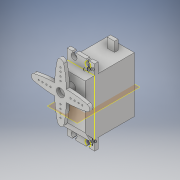
# Autodesk Inventor part: Hew Motor
Saved by Autodesk Inventor 2017 (Build 210142000, 142)
## iProperties
Created: 2016-09-26
Part Number: Hew Motor
Material: Generic
Document SubType Name: Modeling
Designer: situh
Density: 1 g/cm^3
Appearance: Default
Author: situh
Autodesk Inventor part; units mm, degrees
ref_plane "YZ Plane" through (0, 0, 0) normal (1, 0, 0) x (0, 1, 0)
ref_plane "XZ Plane" through (0, 0, 0) normal (0, 1, 0) x (-1, 0, 0)
ref_plane "XY Plane" through (0, 0, 0) normal (0, 0, 1) x (1, 0, 0)
sketch "Sketch1" plane through (0, 0, 0) normal (0, 0, 1) x (1, 0, 0)
  line L0 (-0.8096, 19.4036) -> (19.1904, 19.4036)
  line L1 (19.1904, 19.4036) -> (19.1904, -21.0964)
  line L2 (19.1904, -21.0964) -> (-0.8096, -21.0964)
  line L3 (-0.8096, -21.0964) -> (-0.8096, 19.4036)
  point P0 (0, 0)
  dimension "d0" = 40.5
  dimension "d1" = 20
  constraints: 8 end point, 2 parallel, 1 horizontal, 1 perpendicular
  measures "d0" distance of L0.end L1.end
  measures "d1" distance of L0.start L0.end
extrude "Extrusion1" add sketch "Sketch1" along normal blind 35.9918
sketch "Sketch2" plane through (0, 0, 35.9918) normal (0, 0, 1) x (1, 0, 0)
  circle A0 centre (9.2336, 11.0968) radius 2.9464
  point P0 (0, 0)
  point P1 (-0.8096, -21.0964)
  point P2 (19.1904, -21.0964)
  dimension "d5" = 5.8928
  constraints: 1 centre point
  measures "d5" diameter of A0
extrude "Extrusion2" add sketch "Sketch2" along normal blind 5.6896
sketch "Sketch3" plane through (-0.8096, -21.0964, 0) normal (0, -1, 0) x (1, 0, 0)
  line L0 (0, 0) -> (0, 35.9918) projected
  line L1 (20, 0) -> (20, 35.9918) projected
  line L2 (0, 29.1) -> (20, 29.1)
  line L3 (20, 29.1) -> (20, 26.6)
  line L4 (20, 26.6) -> (0, 26.6)
  line L5 (0, 26.6) -> (0, 29.1)
  point P0 (0.8096, 0)
  dimension "d9" = 2.5
  dimension "d48" = 26.6
  constraints: 8 end point, 2 parallel, 2 point on line, 1 horizontal, 1 perpendicular
  measures "d9" distance of L4.end L2.start
  measures "d48" distance of L3.end L1.start
extrude "Extrusion3" add sketch "Sketch3" along normal blind 7.4168
ref_plane "Work Plane1" through (-0.8096, -0.8464, 35.9918) normal (0, 1, 0) x (1, 0, 0)
sketch "Sketch5" plane through (-0.8096, -21.0964, 29.1) normal (0, 0, 1) x (1, 0, 0)
  arc A0 (5.7377, -6.6011) -> (4.2533, -6.5978) centre (5, -4.572) ccw
  line L0 (0, 0) -> (20, 0) construction
  arc A1 (15.7209, -6.6071) -> (14.2793, -6.6071) centre (15, -4.572) ccw
  line L1 (10, -7.4168) -> (10, 0) construction
  line L2 (20, -7.4168) -> (0, -7.4168) projected
  line L3 (3.7603, -7.4168) -> (4.2533, -6.5978)
  line L4 (5.7377, -6.6011) -> (6.2138, -7.4618)
  line L5 (6.2138, -7.4618) -> (3.7603, -7.4168)
  line L6 (16.1887, -7.4168) -> (13.8117, -7.4176)
  line L7 (13.8117, -7.4176) -> (14.2793, -6.6071)
  line L8 (15.7209, -6.6071) -> (16.1887, -7.4168)
  point P0 (0.8096, 21.0964)
  point P1 (5, -6.731)
  point P2 (15, -6.731)
  dimension "d12" = 4.318
  dimension "d13" = 4.572
  dimension "d15" = 4.318
  dimension "d17" = 5
  dimension "d18" = 5
  dimension "d47" = 10
  constraints: 14 end point, 6 point on circle, 2 centre point, 2 point on line, 1 horizontal alignment, 1 midpoint, 10 other
  measures "d12" diameter of A0
  measures "d13" distance from line of A0.centre L0
  measures "d15" diameter of A1
  measures "d17" distance from line of A1.centre L1
  measures "d18" distance from line of L1 A0.centre
  measures "d47" distance of A0.centre A1.centre
extrude "Extrusion4" cut sketch "Sketch5" against normal up to next
mirror "Mirror1" about plane through (-0.8096, -0.8464, 35.9918) normal (0, 1, 0) of "Extrusion3", "Extrusion4"
chamfer "Chamfer1" distance 7.62 distance2 4.064 1 edges at (9.1904, -21.0964, 35.9918) measured on face at (9.0864, -11.3403, 35.9918)
sketch "Sketch6" plane through (-0.8096, 19.4036, 0) normal (0, 1, 0) x (1, 0, 0)
  line L0 (12.573, -7.1077) -> (7.112, -7.1077)
  line L1 (7.112, -7.1077) -> (7.112, -4.5677)
  line L2 (7.112, -4.5677) -> (12.573, -4.5677)
  line L3 (12.573, -4.5677) -> (12.573, -7.1077)
  line L4 (0, 0) -> (0, -26.6) projected
  point P0 (0.8096, 0)
  dimension "d24" = 5.461
  dimension "d25" = 2.54
  dimension "d26" = 7.112
  constraints: 8 end point, 2 parallel, 1 horizontal, 1 perpendicular
  measures "d24" distance of L0.start L0.end
  measures "d25" distance of L0.end L1.end
  measures "d26" distance between parallel lines of L4 L1
extrude "Extrusion5" add sketch "Sketch6" along normal blind 7.0612
sketch "Sketch7" plane through (9.2336, 11.0968, 41.6814) normal (0, 0, 1) x (1, 0, 0)
  circle A0 centre (0, 0) radius 4.2
  line L0 (-4.2582, 3.0135) -> (-4.2, 0.014)
  circle A1 centre (0, 0) radius 2.9464 projected
  line L1 (0, 0) -> (0, 19) construction
  arc A2 (-2.3283, 19.5394) -> (-4.2582, 3.0135) centre (70.5709, 2.6508) ccw
  line L2 (4.2582, 3.0135) -> (4.2, 0.014)
  arc A3 (2.3283, 19.5394) -> (-2.3283, 19.5394) centre (0, 19) ccw
  arc A4 (4.2582, 3.0135) -> (2.3283, 19.5394) centre (-70.5709, 2.6508) ccw
  circle A5 centre (0, 7.34) radius 0.5
  circle A6 centre (0, 10.25) radius 0.4953
  circle A7 centre (0, 13.24) radius 0.4953
  circle A8 centre (0, 15.97) radius 0.4953
  arc A9 (-19.5394, 2.3283) -> (-19.5394, -2.3283) centre (-19, 0) ccw
  arc A10 (-19.5394, -2.3283) -> (-3.0135, -4.2582) centre (-2.6508, 70.5709) ccw
  arc A11 (-3.0135, 4.2582) -> (-19.5394, 2.3283) centre (-2.6508, -70.5709) ccw
  circle A12 centre (-15.97, 0) radius 0.4953
  circle A13 centre (-13.24, 0) radius 0.4953
  circle A14 centre (-10.25, 0) radius 0.4953
  circle A15 centre (-7.34, 0) radius 0.5
  line L3 (-3.0135, -4.2582) -> (-0.014, -4.2)
  line L4 (-3.0135, 4.2582) -> (-0.014, 4.2)
  circle A16 centre (0, 0) radius 4.2
  arc A17 (-2.3283, -19.5394) -> (2.3283, -19.5394) centre (0, -19) ccw
  arc A18 (2.3283, -19.5394) -> (4.2582, -3.0135) centre (-70.5709, -2.6508) ccw
  arc A19 (-4.2582, -3.0135) -> (-2.3283, -19.5394) centre (70.5709, -2.6508) ccw
  circle A20 centre (0, -15.97) radius 0.4953
  circle A21 centre (0, -13.24) radius 0.4953
  circle A22 centre (0, -10.25) radius 0.4953
  circle A23 centre (0, -7.34) radius 0.5
  line L5 (4.2582, -3.0135) -> (4.2, -0.014)
  line L6 (-4.2582, -3.0135) -> (-4.2, -0.014)
  circle A24 centre (0, 0) radius 4.2
  arc A25 (19.5394, -2.3283) -> (19.5394, 2.3283) centre (19, 0) ccw
  arc A26 (19.5394, 2.3283) -> (3.0135, 4.2582) centre (2.6508, -70.5709) ccw
  arc A27 (3.0135, -4.2582) -> (19.5394, -2.3283) centre (2.6508, 70.5709) ccw
  circle A28 centre (15.97, 0) radius 0.4953
  circle A29 centre (13.24, 0) radius 0.4953
  circle A30 centre (10.25, 0) radius 0.4953
  circle A31 centre (7.34, 0) radius 0.5
  line L7 (3.0135, 4.2582) -> (0.014, 4.2)
  line L8 (3.0135, -4.2582) -> (0.014, -4.2)
  circle A32 centre (0, 0) radius 4.2
  point P0 (-9.2336, -11.0968)
  dimension "d29" = 19
  dimension "d31" = 8.4
  dimension "d33" = 1
  dimension "d34" = 7.34
  dimension "d35" = 0.9906
  dimension "d36" = 10.25
  dimension "d37" = 0.9906
  dimension "d38" = 13.24
  dimension "d39" = 0.9906
  dimension "d40" = 15.97
  dimension "d43" = 360
  constraints: 32 centre point, 32 point on circle, 18 end point, 4 point on line, 3 symmetric about line, 1 coincident, 1 vertical, 98 other
  measures "d29" distance of L1.start L1.end
  measures "d31" diameter of A0
  measures "d33" diameter of A5
  measures "d34" distance of point (0, 0) A5.centre
  measures "d35" diameter of A6
  measures "d36" distance of point (0, 0) A6.centre
  measures "d37" diameter of A7
  measures "d38" distance of point (0, 0) A7.centre
  measures "d39" diameter of A8
  measures "d40" distance of point (0, 0) A8.centre
extrude "Extrusion6" add sketch "Sketch7" along normal blind 2.413
sketch "Sketch9" plane through (-0.8096, 19.4036, 29.1) normal (0, 0, 1) x (1, 0, 0)
  line L0 (20, 0) -> (20, -40.5) projected
  arc A0 (14.2793, 6.6071) -> (15.7209, 6.6071) centre (15, 4.572) ccw projected
  line L1 (15, 4.572) -> (15, 0) construction
  line L2 (0, 0) -> (20, 0) projected
  arc A1 (15.7209, -47.1071) -> (14.2793, -47.1071) centre (15, -45.072) ccw projected
  line L3 (15, -45.072) -> (15, -40.5)
  point P0 (0.8096, -19.4036)
  dimension "d49" = 4.572
  dimension "d50" = 4.572
  constraints: 4 end point, 2 vertical, 1 point on line
  measures "d49" distance of L1.start L1.end
  measures "d50" distance of L3.start L3.end
body "Solid1"
